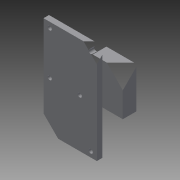
# Autodesk Inventor part: MostekH
Saved by Autodesk Inventor 2015 (Build 190159000, 159)
## iProperties
Created: 2015-05-04
Part Number: MostekH
Material: Ogólny
Document SubType Name: Modeling
Designer: Kuba
Density: 1 g/cm^3
Appearance: Domyślna
Author: Kuba
Autodesk Inventor part; units mm, degrees
ref_plane "YZ Plane" through (0, 0, 0) normal (1, 0, 0) x (0, 1, 0)
ref_plane "XZ Plane" through (0, 0, 0) normal (0, 1, 0) x (-1, 0, 0)
ref_plane "XY Plane" through (0, 0, 0) normal (0, 0, 1) x (1, 0, 0)
sketch "Szkic1" plane through (0, 0, 0) normal (0, 1, 0) x (-1, 0, 0)
  line L0 (-19.5, -35.5) -> (19.5, -35.5)
  line L1 (19.5, -35.5) -> (19.5, 35.5)
  line L2 (19.5, 35.5) -> (-19.5, 35.5)
  line L3 (-19.5, 35.5) -> (-19.5, -35.5)
  line L4 (-19.5, -35.5) -> (19.5, 35.5) construction
  line L5 (19.5, -35.5) -> (-19.5, 35.5) construction
  point P0 (0, 0)
  dimension "d0" = 39
  dimension "d1" = 71
  constraints: 12 end point, 2 midpoint, 2 parallel, 1 horizontal, 1 perpendicular
  measures "d0" distance of L2.end L1.end
  measures "d1" distance of L1.end L0.end
extrude "Wyciągnięcie proste1" add sketch "Szkic1" along normal blind 4
sketch "Szkic2" plane through (0, 4, 0) normal (0, 1, 0) x (1, 0, 0)
  line L0 (19.5, 35.5) -> (-19.5, 35.5) projected
  line L1 (-19.5, 35.5) -> (-19.5, -35.5) projected
  line L2 (-19.5, -35.5) -> (19.5, -35.5) projected
  line L3 (19.5, -35.5) -> (19.5, 35.5) projected
  point P0 (0, 0)
  point P1 (-15, -31.5)
  point P2 (-15, 31.5)
  point P3 (15, 31.5)
  point P4 (15, -31.5)
  point P5 (-15, 0)
  point P6 (7, 0)
  dimension "d4" = 4
  dimension "d5" = 4.5
  dimension "d6" = 63
  dimension "d7" = 63
  dimension "d8" = 71
  dimension "d9" = 4
  dimension "d10" = 30
  dimension "d11" = 39
  dimension "d12" = 30
  dimension "d13" = 4.5
  dimension "d29" = 4.5
  dimension "d30" = 31.5
  dimension "d31" = 22
  measures "d4" distance from line of L2 point (-15, -31.5)
  measures "d5" distance from line of L1 point (-15, -31.5)
  measures "d6" distance of point (-15, 31.5) point (-15, -31.5)
  measures "d7" distance of point (15, -31.5) point (15, 31.5)
  measures "d8" distance of L2.end L0.start
  measures "d9" distance from line of L2 point (15, -31.5)
  measures "d10" distance of point (15, -31.5) point (-15, -31.5)
  measures "d11" distance of L0.start L0.end
  measures "d12" distance of point (15, 31.5) point (-15, 31.5)
  measures "d13" distance from line of L1 point (-15, 31.5)
  measures "d29" distance from line of L1 point (-15, 0)
  measures "d30" distance of point (-15, 31.5) point (-15, 0)
  measures "d31" distance of point (7, 0) point (-15, 0)
hole "Otwór1" at (-15, 4, 31.5) at (-15, 4, -31.5) at (15, 4, -31.5) at (15, 4, 31.5) at (7, 4, 0) at (-15, 4, 0) direction (0, -1, 0) diameter 3 end through all
sketch "Szkic3" plane through (0, 4, 0) normal (0, 1, 0) x (1, 0, 0)
  circle A0 centre (15, 31.5) radius 1.5 projected
  circle A1 centre (-15, -31.5) radius 1.5 projected
  circle A2 centre (-15, 31.5) radius 1.5 projected
  circle A3 centre (15, -31.5) radius 1.5 projected
  line L0 (19.5, 35.5) -> (-19.5, 35.5) projected
  line L1 (-19.5, 35.5) -> (-19.5, -35.5) projected
  line L2 (-19.5, -35.5) -> (19.5, -35.5) projected
  line L3 (19.5, -35.5) -> (19.5, 35.5) projected
  line L4 (12.5, -26.5) -> (19.5, -26.5)
  line L5 (19.5, -26.5) -> (19.5, 3.5)
  line L6 (19.5, 3.5) -> (12.5, 3.5)
  line L7 (12.5, 3.5) -> (12.5, -26.5)
  point P0 (0, 0)
  dimension "d21" = 7
  dimension "d22" = 30
  dimension "d23" = 0
  dimension "d24" = 9
  constraints: 8 end point, 2 parallel, 1 horizontal, 1 perpendicular
  measures "d21" distance of L6.end L5.end
  measures "d22" distance of L5.end L4.end
  measures "d23" distance between parallel lines of L3 L5
  measures "d24" distance between parallel lines of L2 L4
extrude "Wyciągnięcie proste2" add sketch "Szkic3" along normal blind 10 contours L3 L4 L7 L6
sketch "Szkic4" plane through (19.5, 0, 35.5) normal (1, 0, 0) x (0, 0, -1)
  line L0 (0, 0) -> (71, 0) projected
  line L1 (71, 0) -> (71, 4) projected
  line L2 (39, 4) -> (71, 4) projected
  line L3 (39, 4) -> (39, 14) projected
  line L4 (9, 14) -> (39, 14) projected
  line L5 (9, 4) -> (9, 14) projected
  line L6 (0, 4) -> (9, 4) projected
  line L7 (0, 0) -> (0, 4) projected
  line L8 (9, 14) -> (39, 14)
  line L9 (39, 14) -> (39, 4)
  line L10 (39, 4) -> (9, 4)
  line L11 (9, 4) -> (9, 14)
  point P0 (35.5, 0)
  constraints: 8 end point, 2 parallel, 1 horizontal, 1 perpendicular
extrude "Wyciągnięcie proste3" add sketch "Szkic4" along normal blind 15 contours L5 L4 L3 L10
equation "\"d4\" = d9"
equation "\"d5\" = -0.5 * d10 + 0.5 * d11"
equation "\"d9\" = -0.5 * d7 + 0.5 * d8"
equation "\"d12\" = d10"
equation "\"d13\" = d5"
equation "\"d29\" = d13"
equation "\"d30\" = 0.5 * d6"
